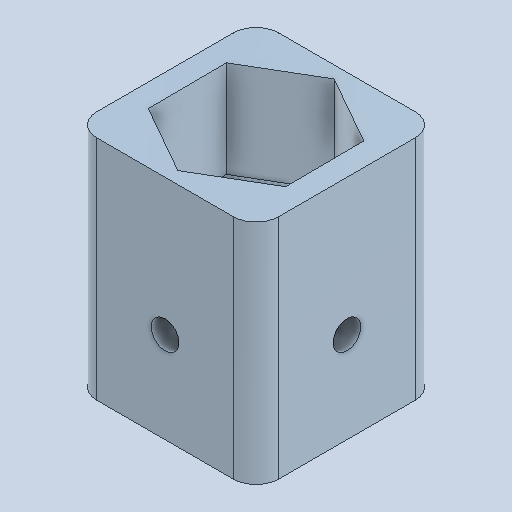
# Autodesk Inventor part: couplingload
Saved by Autodesk Inventor 2025.4 (Build 294407000, 407)
## iProperties
Created: 2026-03-22
Part Number: couplingload
Material: Generic
Document SubType Name: Modeling
Designer: hp
Density: 1 g/cm^3
Appearance: Steel Blue
Author: hp
Autodesk Inventor part; units mm, degrees
ref_plane "YZ Plane" through (0, 0, 0) normal (1, 0, 0) x (0, 1, 0)
ref_plane "XZ Plane" through (0, 0, 0) normal (0, 1, 0) x (-1, 0, 0)
ref_plane "XY Plane" through (0, 0, 0) normal (0, 0, 1) x (1, 0, 0)
sketch "Sketch1" plane through (0, 0, 0) normal (0, 1, 0) x (-1, 0, 0)
  line L0 (0.0535, -6.928) -> (-5.9731, -3.5103)
  line L1 (-5.9731, -3.5103) -> (-6.0266, 3.4177)
  line L2 (-6.0266, 3.4177) -> (-0.0535, 6.928)
  line L3 (-0.0535, 6.928) -> (5.9731, 3.5103)
  line L4 (5.9731, 3.5103) -> (6.0266, -3.4177)
  line L5 (6.0266, -3.4177) -> (0.0535, -6.928)
  line L6 (6, 8) -> (-6, 8)
  line L7 (-8, 6) -> (-8, -6)
  line L8 (-6, -8) -> (6, -8)
  line L9 (8, -6) -> (8, 6)
  line L10 (8, 8) -> (-8, -8) construction
  line L11 (-8, 8) -> (8, -8) construction
  arc A0 (8, 6) -> (6, 8) centre (6, 6) ccw
  arc A1 (-6, 8) -> (-8, 6) centre (-6, 6) ccw
  arc A2 (-8, -6) -> (-6, -8) centre (-6, -6) ccw
  arc A3 (6, -8) -> (8, -6) centre (6, -6) ccw
  point P0 (0, 0)
  point P1 (0, 0)
  dimension "d0" = 12
  dimension "d1" = 16
  dimension "d2" = 16
  dimension "d7" = 2
  constraints: 24 end point, 8 point on circle, 8 point on line, 8 tangent, 4 centre point, 3 equal radius, 2 midpoint, 2 parallel, 1 coincident, 1 horizontal, 1 perpendicular, 13 other
  measures "d0" distance between parallel lines of L1 L4
  measures "d1" distance of L11.end L10.end
  measures "d2" distance of L10.end L11.start
  measures "d7" radius of A0
extrude "Extrusion1" add sketch "Sketch1" along normal blind 8.5
extrude "Extrusion2" add sketch "Sketch1" against normal blind 11.5 contours L0 L1 L2 L3 L4 L5 | A0 L9 A3 L8 A2 L7 A1 L6
sketch "Sketch2" plane through (8, 8.5, 6) normal (1, 0, 0) x (0, 0, -1)
  line L0 (12, -20) -> (12, 0) projected
  line L1 (0, 0) -> (12, 0) projected
  line L2 (0, -20) -> (0, 0) projected
  line L3 (12, -20) -> (0, -20) projected
  point P0 (6, -8.5)
  point P1 (6, -12)
  point P2 (6, -20)
  dimension "d8" = 12
  constraints: 1 midpoint
  measures "d8" distance from line of point (6, -12) L1
hole "Hole1" at (8, -3.5, 0) direction (-1, 0, 0) diameter 2.45 depth 3 tip angle 118
pattern_circular "Circular Pattern1" count 4 over 360 about axis through (0, -10, 0) along (0, 1, 0) of "Hole1"
body "Solid1"
